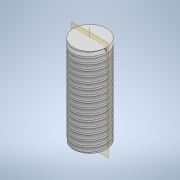
# Autodesk Inventor part: threadExample
Saved by Autodesk Inventor 2021 (Build 250183000, 183)
## iProperties
Created: 2020-06-13
Part Number: threadExample
Material: Generic
Document SubType Name: Modeling
Designer: robst
Density: 1 g/cm^3
Appearance: Default
Author: robst
Autodesk Inventor part; units mm, degrees
ref_plane "YZ Plane" through (0, 0, 0) normal (1, 0, 0) x (0, 1, 0)
ref_plane "XZ Plane" through (0, 0, 0) normal (0, 1, 0) x (-1, 0, 0)
sketch "Sketch1" plane through (0, 0, 0) normal (0, 1, 0) x (-1, 0, 0)
  circle A0 centre (0, 0) radius 4.746
  dimension "d0" = 9.492
  constraints: 1 centre point, 1 coincident
  measures "d0" diameter of A0
extrude "Extrusion1" add sketch "Sketch1" against normal blind 25.4
sketch "Sketch11" plane through (0, 0, 0) normal (0, 0, 1) x (1, 0, 0)
  line L0 (4.746, 0) -> (4.746, -25.4) projected
  line L1 (-4.746, -25.4) -> (4.746, -25.4) projected
  line L2 (4.746, -25.4) -> (3.7998, -25.9463)
  line L3 (0, -31.791) -> (0, 5.2985) projected
  line L4 (3.7998, -25.9463) -> (4.746, -26.4925)
  line L5 (4.746, -26.4925) -> (4.746, -25.4)
  point P0 (0, 0)
  dimension "d118" = 30
  dimension "d119" = 3.7998
  dimension "d128" = 4.746
  constraints: 6 end point, 1 collinear, 1 equal length, 1 point on line
  measures "d118" angle of L2 L1
  measures "d119" distance from line of L2.end L3
  measures "d128" distance between parallel lines of L5 L3
coil "Coil12" sketch "Sketch11" operation cut axis through (0, -10, 0) along (0, 1, 0) pitch 1.5875 turns 16 hand right
body "Solid1"
